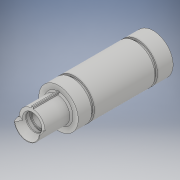
# Autodesk Inventor part: douille_bloqueur
Saved by Autodesk Inventor 2019 (Build 230136000, 136)
## iProperties
Created: 2019-03-19
Part Number: douille_bloqueur
Material: Générique
Document SubType Name: Modeling
Designer: theor
Density: 1 g/cm^3
Appearance: Par défaut
Mass: 45.3835 g
Surface Area: 244.644 cm^2
Volume: 45.3835 cm^3
Author: theor
Autodesk Inventor part; units mm, degrees
ref_plane "YZ Plane" through (0, 0, 0) normal (1, 0, 0) x (0, 1, 0)
ref_plane "XZ Plane" through (0, 0, 0) normal (0, 1, 0) x (-1, 0, 0)
ref_plane "XY Plane" through (0, 0, 0) normal (0, 0, 1) x (1, 0, 0)
sketch "Esquisse1" plane through (0, 0, 0) normal (1, 0, 0) x (0, 1, 0)
  line L0 (0, 0) -> (0, -31.2712)
  line L1 (18.75, -30) -> (18.75, -120)
  line L2 (18.75, -120) -> (0, -120)
  line L3 (14.75, -116) -> (14.75, -55.9524)
  line L4 (14.75, -55.9524) -> (7, -12)
  line L5 (7, -12) -> (7, -11)
  line L6 (7, -11) -> (8, -11)
  line L7 (8, -11) -> (9.7, -12.2)
  line L8 (9.7, -12.2) -> (10.85, -8.8246)
  line L9 (10.85, -8.8246) -> (8.25, -8)
  circle A0 centre (8.85, -9.7639) radius 1.5 construction
  line L10 (8.25, -8) -> (8.25, -7)
  line L11 (8.25, -7) -> (11.75, 0)
  line L12 (18.75, -30) -> (12.25, -30)
  line L13 (12.25, -30) -> (12.25, 0)
  line L14 (12.25, 0) -> (11.75, 0)
  line L15 (0, -120) -> (0, -116)
  line L16 (14.75, -116) -> (0, -116)
  point P0 (9.7477, -27.583)
  dimension "d1" = 37.5
  dimension "d3" = 14
  dimension "d6" = 3
  dimension "d7" = 1
  dimension "d8" = 1
  dimension "d11" = 3
  dimension "d12" = 0.6
  dimension "d13" = 1.2
  dimension "d14" = 1.7
  dimension "d15" = 2.6
  dimension "d29" = 24.5
  dimension "d30" = 0.5
  dimension "d31" = 30
  dimension "d34" = 1
  dimension "d36" = 16.5
  dimension "d37" = 11
  dimension "d38" = 90
  dimension "d58" = 7.75
  dimension "d59" = 170
  dimension "d60" = 19.4954
  dimension "d61" = 4
  dimension "d62" = 4
  constraints: 34 end point, 7 vertical, 5 horizontal, 2 tangent, 1 centre point, 1 collinear, 1 horizontal alignment, 1 point on line
  measures "d1" diameter of L1 L0
  measures "d3" diameter of L4.end L0
  measures "d6" diameter of A0
  measures "d7" distance of L4.end L5.end
  measures "d8" distance of L5.end L6.end
  measures "d11" vertical distance of L9.end L6.end
  measures "d12" horizontal distance of L9.end A0.centre
  measures "d13" vertical distance of L6.end L7.end
  measures "d14" horizontal distance of L6.end L7.end
  measures "d15" horizontal distance of L8.end L9.end
  measures "d29" diameter of L13 L0
  measures "d30" distance of L13.end L11.end
  measures "d31" distance between parallel lines of L14 L12
  measures "d34" distance of L9.end L10.end
  measures "d36" diameter of L10 L0
  measures "d37" vertical distance of L11.end L5.end
  measures "d38" distance between parallel lines of L2 L12
  measures "d58" horizontal distance of L3.end L4.end
  measures "d59" angle of L3 L4
  measures "d60" diameter of point (9.748, -27.583) L0
  measures "d61" distance between parallel lines of L1 L3
  measures "d62" distance of L2.end L15.end
revolve "Révolution2" add sketch "Esquisse1" angle 360 about axis through (0, 0, 0) along (0, 0, -1)
sketch "Esquisse2" plane through (0, 0, 0) normal (0, 1, 0) x (-1, 0, 0)
  line L0 (-18.75, -30) -> (18.75, -30) projected
  line L1 (-18.75, -120) -> (18.75, -120) projected
  line L2 (-14.75, -55.9524) -> (14.75, -55.9524) projected
  line L3 (-7, -12) -> (7, -12) projected
  line L4 (-18.75, -30) -> (-18.75, -120) projected
  line L5 (-18.75, -42.7677) -> (-16.25, -41.8578)
  line L6 (-16.25, -41.8578) -> (-16.25, -46.1422)
  line L7 (-16.25, -46.1422) -> (-18.75, -45.2323)
  circle A0 centre (-17.75, -44) radius 1.5 construction
  line L8 (0, -144) -> (0, 24) projected
  point P0 (0, 0)
  dimension "d42" = 3
  dimension "d45" = 1
  dimension "d46" = 70
  dimension "d47" = 70
  dimension "d48" = 14
  constraints: 6 end point, 3 tangent, 2 point on line, 1 centre point, 1 vertical
  measures "d42" diameter of A0
  measures "d45" distance from line of L4 A0.centre
  measures "d46" angle of L6 L7
  measures "d47" angle of L6 L5
  measures "d48" distance from line of A0.centre L0
revolve "Révolution3" cut sketch "Esquisse2" angle 360 about axis through (0, 0, -10) along (0, 0, 1) contours L5 L6 L7 L4
chamfer "Chanfrein4" distance 1.5 angle 45 1 edges at (0, -12.25, -30)
pattern_linear "Réseau rectangulaire1" count 2 spacing 60 along (0, 0, -1) of "Révolution3"
chamfer "Chanfrein5" distance 2 angle 45 1 edges at (0, -14.75, -116)
sketch "Esquisse3" plane through (0, 0, 0) normal (0, 0, 1) x (1, 0, 0)
  circle A0 centre (0, 0) radius 11.75 projected
  circle A1 centre (0, 0) radius 12.25 projected
  line L0 (-1, 14.2091) -> (1, 14.2091)
  line L1 (1, 14.2091) -> (1, 12.2091)
  line L2 (1, 12.2091) -> (-1, 12.2091)
  line L3 (-1, 12.2091) -> (-1, 14.2091)
  circle A2 centre (0, 0) radius 12.25 projected
  point P0 (0, 12.2091)
  dimension "d66" = 2
  dimension "d67" = 2
  constraints: 8 end point, 2 parallel, 1 horizontal, 1 midpoint, 1 perpendicular, 1 vertical alignment, 2 other
  measures "d66" distance of L0.start L0.end
  measures "d67" distance of L0.end L1.end
extrude "Extrusion1" add sketch "Esquisse3" against normal up to surface (30 mm away) contours L2 A1 | A1 L3 L0 L1 picked at (-0.1112, 12.2212)
chamfer "Chanfrein6" distance 0.5 angle 45 2 edges at (1, 14.2091, -15) (-1, 14.2091, -15)
sketch "Esquisse8" plane through (0, 0, -120) normal (0, 0, -1) x (-1, 0, 0)
  circle A0 centre (0, 0) radius 5
  dimension "d100" = 10
  constraints: 1 centre point, 1 coincident
  measures "d100" diameter of A0
extrude "Extrusion5" cut sketch "Esquisse8" against normal up to surface (4 mm away)
chamfer "Chanfrein8" distance 1 angle 45 2 edges at (5, 0, -120) (5, 0, -116)
sketch "Esquisse9" plane through (0, 0, 0) normal (0, 1, 0) x (-1, 0, 0)
  line L0 (1, 0) -> (1, -28.5) projected
  line L1 (-1, -28.5) -> (1, -28.5) projected
  line L2 (-1, -28.5) -> (-1, 0) projected
  line L3 (-1, 0) -> (1, 0) projected
  line L4 (8.25, -7) -> (11.75, 0) projected
  line L5 (-8.25, -7) -> (-11.75, 0) projected
  line L6 (12.25, 0) -> (-12.25, 0)
  line L7 (-12.25, 0) -> (-12.25, -5)
  line L8 (-12.25, -5) -> (12.25, -5)
  line L9 (12.25, -5) -> (12.25, 0)
  line L10 (-12.25, 0) -> (12.25, 0) projected
  line L11 (-8.25, -7) -> (8.25, -7) projected
  line L12 (-12.25, 0) -> (-12.25, -28.5) projected
  point P0 (0, 0)
  dimension "d108" = 2
  dimension "d112" = 5
  constraints: 8 end point, 2 parallel, 1 horizontal, 1 perpendicular, 1 point on line
  measures "d108" distance between parallel lines of L11 L8
  measures "d112" distance of L6.end L7.end
extrude "Extrusion6" cut sketch "Esquisse9" along normal blind 15 contours L6 L4 L8 L0 | L0 L8 L2 L3 | L2 L8 L5 L6 | L6 L9 L8 L4 | L5 L8 L7 L6
chamfer "Chanfrein9" distance 2 angle 45 2 edges at (10.5, 0, -2.5) (-10.5, 0, -2.5)
equation "\"d47\" = d46"
